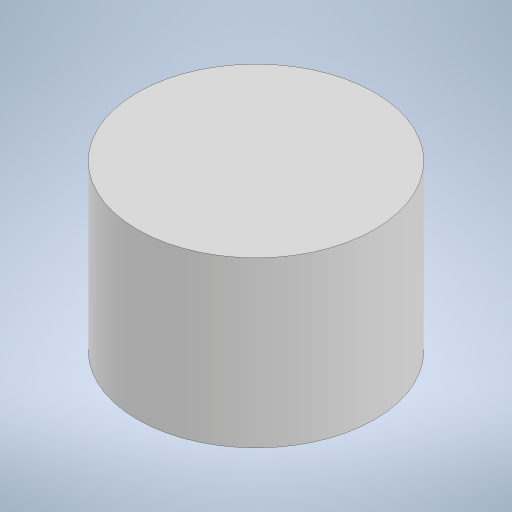
# Autodesk Inventor part: Multiboard Thread insert
Saved by Autodesk Inventor 2024.3 (Build 283343000, 343)
## iProperties
Created: 2024-11-06
Part Number: Multiboard Thread insert
Material: Generic
Document SubType Name: Modeling
Designer: wszaf
Density: 1 g/cm^3
Appearance: Default
Author: wszaf
Autodesk Inventor part; units mm, degrees
ref_plane "YZ Plane" through (0, 0, 0) normal (1, 0, 0) x (0, 1, 0)
ref_plane "XZ Plane" through (0, 0, 0) normal (0, 1, 0) x (-1, 0, 0)
ref_plane "XY Plane" through (0, 0, 0) normal (0, 0, 1) x (1, 0, 0)
sketch "Sketch4" plane through (0, 0, 0) normal (0, 1, 0) x (-1, 0, 0)
  circle A0 centre (0, 0) radius 3.05
  circle A1 centre (0, 0) radius 5
  circle A2 centre (-12.0305, -0.1757) radius 3.05
  circle A3 centre (-12.0305, -0.1757) radius 5
  circle A4 centre (-21.0308, 0) radius 3.1
  dimension "d13" = 6.1
  dimension "d14" = 10
  dimension "d25" = 6.1
  dimension "d26" = 10
  dimension "d30" = 6.2
  constraints: 5 centre point, 4 coincident
  measures "d13" diameter of A0
  measures "d14" diameter of A1
  measures "d25" diameter of A2
  measures "d26" diameter of A3
  measures "d30" diameter of A4
extrude "Extrusion5" add sketch "Sketch4" along normal blind 2.5 contours A0 | A1 | A2 | A3
extrude "Extrusion6" cut sketch "Sketch4" along normal blind 2.1 contours A0 | A2
sketch "Sketch5" plane through (0, 2.5, 0) normal (0, 1, 0) x (1, 0, 0)
  circle A0 centre (0, 0) radius 3.8
  dimension "d19" = 7.6
  constraints: 1 centre point, 1 coincident
  measures "d19" diameter of A0
extrude "Extrusion7" add sketch "Sketch5" along normal blind 7.2
sketch "Sketch6" plane through (0, 9.7, 0) normal (0, 1, 0) x (1, 0, 0)
  circle A0 centre (0, 0) radius 3
  dimension "d22" = 6
  constraints: 1 centre point, 1 coincident
  measures "d22" diameter of A0
extrude "Extrusion8" cut sketch "Sketch6" against normal blind 4.2
sketch "Sketch7" plane through (12.0305, 2.5, -0.1757) normal (0, 1, 0) x (1, 0, 0)
  circle A0 centre (0, 0) radius 3.1
  circle A1 centre (0, 0) radius 5 projected
  point P0 (-12.0305, -0.1757)
  dimension "d27" = 6.2
  constraints: 1 centre point, 1 concentric
  measures "d27" diameter of A0
extrude "Extrusion9" add sketch "Sketch7" along normal blind 4 contours A0
extrude "Extrusion10" add sketch "Sketch4" along normal blind 4.3 contours A4
sketch "Sketch8" plane through (0, 0, 0) normal (0, 1, 0) x (-1, 0, 0)
  circle A0 centre (0, 0) radius 3.05 projected
  circle A1 centre (0, 0) radius 5 projected
  circle A2 centre (-12.0305, -0.1757) radius 5 projected
split body "Split1" sketch "Sketch8" result two bodies curves A1 first body at (3.2893, 7.3, 0.2655)
split body "Split2" sketch "Sketch8" result two bodies bodies 3 curves A2 first body at (7.5887, 1.6667, -0.8976)
equation "\"d19\" = Shaft_Diameter - Shaft_Fit_Loose"
equation "\"Shaft_Diameter\" = 8"
equation "\"Shaft_Fit_Loose\" = 0.4"
equation "\"Shaft_Width\" = 7"
equation "\"Distance_Between\" = 3"
